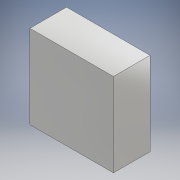
# Autodesk Inventor part: MAGNET
Saved by Autodesk Inventor 2017.3 (Build 213256000, 256)
## iProperties
Created: 2018-01-04
Part Number: MAGNET
Material: Generic
Document SubType Name: Modeling
Designer: Alex
Density: 1 g/cm^3
Appearance: Aluminum - Polished
magnet_A: 5,350 mm
magnet_B: 2,350 mm
Author: Alex
Autodesk Inventor part; units mm, degrees
ref_plane "YZ Plane" through (0, 0, 0) normal (1, 0, 0) x (0, 1, 0)
ref_plane "XZ Plane" through (0, 0, 0) normal (0, 1, 0) x (-1, 0, 0)
ref_plane "XY Plane" through (0, 0, 0) normal (0, 0, 1) x (1, 0, 0)
sketch "Sketch1" plane through (0, 0, 0) normal (0, 1, 0) x (-1, 0, 0)
  line L0 (-2.675, 2.675) -> (2.675, 2.675)
  line L1 (2.675, 2.675) -> (2.675, -2.675)
  line L2 (2.675, -2.675) -> (-2.675, -2.675)
  line L3 (-2.675, -2.675) -> (-2.675, 2.675)
  point P0 (0, 0)
  point P1 (0, -2.675)
  point P2 (2.675, 0)
  dimension "d0" = 5.35
  constraints: 8 end point, 2 midpoint, 2 parallel, 2 perpendicular, 1 horizontal, 1 horizontal alignment, 1 vertical alignment
  measures "d0" distance of L0.end L1.end
extrude "Extrusion1" add sketch "Sketch1" along normal blind 2.35
equation "\"d0\" = magnet_A"
equation "\"d1\" = magnet_B"
equation "\"magnet_A\" = 5.35"
equation "\"magnet_B\" = 2.35"
body "Solid1"
